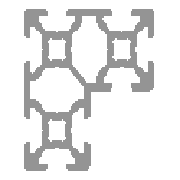
# Autodesk Inventor part: 3 842 992 991-2mm
Saved by Autodesk Inventor 2011 SP1 (Build 150282100, 282)
## iProperties
Created: 2011-02-10
Part Number: 3 842 992 991-2mm
Document SubType Name: Modeling
Designer: S. Wile
Density: 2.71 g/cm^3
Categories: <MemberInstance><Categories><Category DisplayName="Structural Shapes" InternalName="089c4875-fa83-4c05-b084-43b9cc11f5ed" Mnemonic="GRDR"><CategoryParameter DisplayName="Custom Base Point" InternalName="4f1d1b73-316d-484b-a3df-9cbabb16eb77" Mnemonic="shpBasePoint"/><CategoryParameter DisplayName="FG Authored" InternalName="9c666724-f362-4ea7-ac62-f6a007de5c69" Mnemonic="shpFGAuto"/><CategoryParameter DisplayName="Legacy Member ID" InternalName="340afe4f-75d7-48d3-ab7d-943f3c3da468" Mnemonic="LegacyMemberID"/><CategoryParameter DisplayName="Base Length" InternalName="42e34263-8f20-4d0e-ad48-bf1385b87c24" Mnemonic="shplen"/><CategoryParameter DisplayName="Distance of the Center of Gravity X-X" InternalName="26c9bdb8-9c79-4b4f-a92e-8e197583c9c4" Mnemonic="grcendistX"/><CategoryParameter DisplayName="Distance of the Center of Gravity Y-Y" InternalName="bcc4fb17-7af4-436a-8f8c-d0aa3b0248c5" Mnemonic="grcendistY"/><CategoryParameter DisplayName="Torsional Rigidity Modulus" InternalName="26c1ec35-5026-4c63-ad0a-751cf684a536" Mnemonic="torrigmod"/><CategoryParameter DisplayName="Torsional Section Modulus" InternalName="7c55a8dc-8844-49f9-a867-cc677b30ec9a" Mnemonic="torsecmod"/><CategoryParameter DisplayName="Coefficient of Shear Displacement" InternalName="de4c90c6-aaa8-468f-a335-6737b311b5d3" Mnemonic="shdispc"/><CategoryParameter DisplayName="Section Area" InternalName="1ff91680-64b0-4202-b9a3-7fd3f94bba3b" Mnemonic="secarea"/><CategoryParameter DisplayName="Moment of Inertia (x)" InternalName="4cd780bc-73d7-43ac-917a-579e5cbd684d" Mnemonic="inermomx"/><CategoryParameter DisplayName="Moment of Inertia (y)" InternalName="4b9f58ea-bced-460e-81ea-3d29ca5a49e3" Mnemonic="inermomy"/><CategoryParameter DisplayName="Section Module (x)" InternalName="72cfad18-cf51-4ed4-aaa7-c6b224f8419f" Mnemonic="secmodx"/><CategoryParameter DisplayName="Section Module (y)" InternalName="59eaa5e9-d227-48dc-b6c1-6920f96e0f95" Mnemonic="secmody"/><CategoryParameter DisplayName="Radius of Gyration (x)" InternalName="25778675-03e9-40c1-b6a8-4a9ed693320d" Mnemonic="gyrradx"/><CategoryParameter DisplayName="Radius of Gyration (y)" InternalName="bfa18ebe-1636-4dbe-8d42-b263e0b73184" Mnemonic="gyrrady"/><CategoryParameter DisplayName="Shape Thickness" InternalName="d109cf76-8eb4-42fc-9800-4409734adc67" Mnemonic="shpthick"/><CategoryParameter DisplayName="Second Shape Thickness" InternalName="9251a8e1-85fd-4e47-af99-afdb762317d9" Mnemonic="shpthick2"/><CategoryParameter DisplayName="Shape Width" InternalName="7c717d54-a18f-4666-b4d4-573cce22c62c" Mnemonic="shpwdth"/><CategoryParameter DisplayName="Shape Height" InternalName="50274e7d-5ac0-4796-92cb-c59e54983c67" Mnemonic="shpheig"/><CategoryParameter DisplayName="Mass per Length Unit" InternalName="0bb95a10-148f-4027-a459-38d7b056702a" Mnemonic="shpmass"/><CategoryParameter DisplayName="Section Designation" InternalName="5a64d034-428d-49c8-ba32-7619764de20f" Mnemonic="shpdes"/><Category DisplayName="Other" InternalName="f02205ff-2390-476f-921c-0b3185f88e84" Mnemonic="OTHSHP"><CategoryParameter DisplayName="Moment of Inertia (x)" InternalName="ec6737bc-264f-43ed-b0bd-f6d410c2718d" Mnemonic="inermomx"/><CategoryParameter DisplayName="Moment of Inertia (y)" InternalName="044c654e-f649-48ac-84cc-650a29ae31ca" Mnemonic="inermomy"/><CategoryParameter DisplayName="Section Module (x)" InternalName="cac70804-9d39-43bb-be17-56ea1f39a6c2" Mnemonic="secmodx"/><CategoryParameter DisplayName="Section Module (y)" InternalName="88b8bff9-a616-4028-93d5-ed4f79680d13" Mnemonic="secmody"/><CategoryParameter DisplayName="Section Area" InternalName="c46ecdf8-b6eb-4db9-8b25-30258930c1e3" Mnemonic="secarea"/><CategoryParameter DisplayName="Radius of Gyration (x)" InternalName="ee72c61e-565e-4fd6-b448-66e1e1abcb7e" Mnemonic="gyrradx"/><CategoryParameter DisplayName="Radius of Gyration (y)" InternalName="743e1dfe-1bba-408b-b985-cf752b207386" Mnemonic="gyrrady"/><CategoryParameter DisplayName="Shape Thickness" InternalName="12b1a788-9233-48fd-a933-2df8ff42b15f" Mnemonic="shpthick"/><CategoryParameter DisplayName="Mass per Length Unit" InternalName="2fd289d6-9394-4d2d-97e6-6659d7d4551d" Mnemonic="shpmass"/></Category></Category></Categories><FamilyTemplate Id="20x40x40"><FamilyTemplateParameters><FamilyTemplateParameter ObjectType="kUserParameterObject" ValueType="xs:double" Id="1" ObjectReferenceKey="G_L"/><FamilyTemplateParameter ObjectType="kUserParameterObject" ValueType="xs:double" Id="2" ObjectReferenceKey="G_OFFSET_END"/><FamilyTemplateParameter ObjectType="kUserParameterObject" ValueType="xs:double" Id="3" ObjectReferenceKey="G_OFFSET_START"/><FamilyTemplateParameter ObjectType="kUserParameterObject" ValueType="xs:double" Id="4" ObjectReferenceKey="Length"/><FamilyTemplateParameter ObjectType="kPropertyObject" ValueType="xs:string" Id="7" ObjectReferenceKey="{32853F0F-3444-11d1-9E93-0060B03C1CA6}" SubObjectId="52"/><FamilyTemplateParameter ObjectType="kPartComponentDefinitionObject" ValueType="xs:string" Id="8" SubObjectId="Material"/><FamilyTemplateParameter ObjectType="kPropertyObject" ValueType="xs:string" Id="9" ObjectReferenceKey="{32853F0F-3444-11d1-9E93-0060B03C1CA6}" SubObjectId="5"/><FamilyTemplateParameter ObjectType="kPropertyObject" ValueType="xs:string" Id="10" ObjectReferenceKey="{32853F0F-3444-11D1-9E93-0060B03C1CA6}" SubObjectId="55"/><FamilyTemplateParameter ObjectType="kiPartTableColumnObject" ValueType="xs:string" Id="21" ObjectReferenceKey="FILENAME"/><FamilyTemplateParameter ObjectType="kiPartTableColumnObject" ValueType="xs:string" Id="22" ObjectReferenceKey="MEMBER_REVISION"/></FamilyTemplateParameters></FamilyTemplate><CategoryParameterMap><ParamToTemplateMap><ParamToTemplate CategoryParameter="//CategoryParameter[@InternalName='4f1d1b73-316d-484b-a3df-9cbabb16eb77']" ConstantValue="1"/><ParamToTemplate CategoryParameter="//CategoryParameter[@InternalName='9c666724-f362-4ea7-ac62-f6a007de5c69']" ConstantValue="1"/><ParamToTemplate CategoryParameter="//CategoryParameter[@InternalName='2675968c-4ce5-49e0-a4f5-552d29089031']" TemplateParameter="7"/><ParamToTemplate CategoryParameter="//CategoryParameter[@InternalName='8b46a4cc-9585-4fed-90c3-899f57e09a73']" TemplateParameter="21"/><ParamToTemplate CategoryParameter="//CategoryParameter[@InternalName='42e34263-8f20-4d0e-ad48-bf1385b87c24']" TemplateParameter="4"/><ParamToTemplate CategoryParameter="//CategoryParameter[@InternalName='818a152a-d3c3-49ca-80ee-df7d91421b8e']" TemplateParameter="8"/><ParamToTemplate CategoryParameter="//CategoryParameter[@InternalName='a65d44b9-392f-4f4f-857b-e4b3d54996fe']" TemplateParameter="22"/><ParamToTemplate CategoryParameter="//CategoryParameter[@InternalName='016b6077-bfbe-49bd-92c9-d8d59c39c941']" TemplateParameter="9"/></ParamToTemplateMap></CategoryParameterMap></MemberInstance>
Stock Number: 3 842 992 991
Description: PROFILE 20x40x40, -/-
Material: Aluminum-6061
Mass: 2.24182 g
Surface Area: 17.6618 cm^2
Volume: 0.827241 cm^3
Author: S. Wile
Autodesk Inventor part; units mm, degrees
(part 1 of 2)
ref_plane "YZ Plane" through (0, 0, 0) normal (1, 0, 0) x (0, 1, 0)
ref_plane "XZ Plane" through (0, 0, 0) normal (0, 1, 0) x (-1, 0, 0)
ref_plane "XY Plane" through (0, 0, 0) normal (0, 0, 1) x (1, 0, 0)
sketch "20x40x40" plane through (0, 0, 0) normal (0, 0, 1) x (1, 0, 0)
  arc A0 (64.9127, 49.9559) -> (64.8824, 50.1695) centre (64.7308, 50.0391) ccw
  arc A1 (64.9127, 49.9559) -> (64.9127, 47.6687) centre (67.4136, 48.8123) ccw
  arc A2 (55.9136, 39.0445) -> (55.7672, 39.3981) centre (55.4136, 39.0445) ccw
  line L0 (50.9994, 44.1658) -> (55.7672, 39.3981)
  arc A3 (50.9994, 44.1658) -> (50.6458, 44.3123) centre (50.6458, 43.8123) ccw
  line L1 (48.3672, 44.3123) -> (50.6458, 44.3123)
  arc A4 (48.2672, 44.3391) -> (48.3672, 44.3123) centre (48.3672, 44.5123) ccw
  line L2 (47.5136, 44.7742) -> (48.2672, 44.3391)
  arc A5 (47.5136, 44.7742) -> (47.3136, 44.7742) centre (47.4136, 44.601) ccw
  line L3 (46.56, 44.3391) -> (47.3136, 44.7742)
  arc A6 (46.46, 44.3123) -> (46.56, 44.3391) centre (46.46, 44.5123) ccw
  line L4 (44.1814, 44.3123) -> (46.46, 44.3123)
  arc A7 (44.1814, 44.3123) -> (43.8278, 44.1658) centre (44.1814, 43.8123) ccw
  line L5 (43.8278, 44.1658) -> (41.5601, 41.8981)
  arc A8 (40.1458, 41.3123) -> (41.5601, 41.8981) centre (40.1458, 43.3123) ccw
  line L6 (40.1458, 41.3123) -> (39.4136, 41.3123)
  arc A9 (39.4136, 41.3123) -> (38.9136, 40.8123) centre (39.4136, 40.8123) ccw
  line L7 (38.9136, 36.8123) -> (38.9136, 40.8123)
  arc A10 (38.9136, 36.8123) -> (39.4136, 36.3123) centre (39.4136, 36.8123) ccw
  line L8 (40.1458, 36.3123) -> (39.4136, 36.3123)
  arc A11 (41.5601, 35.7265) -> (40.1458, 36.3123) centre (40.1458, 34.3123) ccw
  line L9 (43.8278, 33.4587) -> (41.5601, 35.7265)
  arc A12 (43.8278, 33.4587) -> (44.1814, 33.3123) centre (44.1814, 33.8123) ccw
  line L10 (46.46, 33.3123) -> (44.1814, 33.3123)
  arc A13 (46.56, 33.2855) -> (46.46, 33.3123) centre (46.46, 33.1123) ccw
  line L11 (47.3136, 32.8504) -> (46.56, 33.2855)
  arc A14 (47.3136, 32.8504) -> (47.5136, 32.8504) centre (47.4136, 33.0236) ccw
  line L12 (48.2672, 33.2855) -> (47.5136, 32.8504)
  arc A15 (48.3672, 33.3123) -> (48.2672, 33.2855) centre (48.3672, 33.1123) ccw
  line L13 (50.6458, 33.3123) -> (48.3672, 33.3123)
  arc A16 (50.6458, 33.3123) -> (50.9994, 33.4587) centre (50.6458, 33.8123) ccw
  line L14 (53.2672, 35.7265) -> (50.9994, 33.4587)
  arc A17 (54.6814, 36.3123) -> (53.2672, 35.7265) centre (54.6814, 34.3123) ccw
  line L15 (54.6814, 36.3123) -> (55.4136, 36.3123)
  arc A18 (55.4136, 36.3123) -> (55.9136, 36.8123) centre (55.4136, 36.8123) ccw
  line L16 (49.9395, 50.1746) -> (50.3052, 50.6129)
  arc A19 (50.3052, 50.6129) -> (50.3152, 50.8562) centre (50.1517, 50.741) ccw
  arc A20 (50.3152, 50.8562) -> (49.4575, 51.7138) centre (47.4136, 48.8123) ccw
  arc A21 (49.4575, 51.7138) -> (49.2142, 51.7039) centre (49.3423, 51.5503) ccw
  line L17 (48.7759, 51.3382) -> (49.2142, 51.7039)
  arc A22 (48.5641, 51.3101) -> (48.7759, 51.3382) centre (48.6478, 51.4917) ccw
  arc A23 (48.5641, 51.3101) -> (46.2631, 51.3101) centre (47.4136, 48.8123) ccw
  arc A24 (46.0513, 51.3382) -> (46.2631, 51.3101) centre (46.1795, 51.4917) ccw
  line L18 (46.0513, 51.3382) -> (45.613, 51.7039)
  arc A25 (45.613, 51.7039) -> (45.3697, 51.7138) centre (45.4849, 51.5503) ccw
  arc A26 (45.3697, 51.7138) -> (44.5121, 50.8562) centre (47.4136, 48.8123) ccw
  arc A27 (44.5121, 50.8562) -> (44.5224, 50.6125) centre (44.6756, 50.741) ccw
  line L19 (44.5224, 50.6125) -> (44.8893, 50.1752)
  arc A28 (44.9267, 49.9861) -> (44.8893, 50.1752) centre (44.7361, 50.0466) ccw
  arc A29 (44.9267, 49.9861) -> (44.9165, 47.6603) centre (47.4136, 48.8123) ccw
  arc A30 (44.8893, 47.4494) -> (44.9165, 47.6603) centre (44.7349, 47.5765) ccw
  line L20 (44.5224, 47.0121) -> (44.8893, 47.4494)
  arc A31 (44.5224, 47.0121) -> (44.5121, 46.7684) centre (44.6756, 46.8836) ccw
  arc A32 (44.5121, 46.7684) -> (45.3777, 45.9051) centre (47.4136, 48.8123) ccw
  arc A33 (45.3777, 45.9051) -> (45.621, 45.9158) centre (45.4924, 46.069) ccw
  line L21 (45.621, 45.9158) -> (46.0582, 46.2827)
  arc A34 (46.27, 46.3114) -> (46.0582, 46.2827) centre (46.1868, 46.1295) ccw
  arc A35 (46.27, 46.3114) -> (48.5641, 46.3145) centre (47.4136, 48.8123) ccw
  arc A36 (48.7759, 46.2864) -> (48.5641, 46.3145) centre (48.6478, 46.1329) ccw
  line L22 (48.7759, 46.2864) -> (49.2142, 45.9207)
  arc A37 (49.2142, 45.9207) -> (49.4575, 45.9107) centre (49.3423, 46.0742) ccw
  arc A38 (49.4575, 45.9107) -> (50.3152, 46.7684) centre (47.4136, 48.8123) ccw
  arc A39 (50.3152, 46.7684) -> (50.3052, 47.0117) centre (50.1517, 46.8836) ccw
  line L23 (50.3052, 47.0117) -> (49.9395, 47.45)
  arc A40 (49.9114, 47.6618) -> (49.9395, 47.45) centre (50.093, 47.5781) ccw
  arc A41 (49.9114, 47.6618) -> (49.9114, 49.9628) centre (47.4136, 48.8123) ccw
  line L24 (46.0513, 31.3382) -> (45.613, 31.7039)
  arc A42 (45.613, 31.7039) -> (45.3697, 31.7138) centre (45.4849, 31.5503) ccw
  arc A43 (45.3697, 31.7138) -> (44.5121, 30.8562) centre (47.4136, 28.8123) ccw
  arc A44 (44.5121, 30.8562) -> (44.522, 30.6129) centre (44.6756, 30.741) ccw
  line L25 (44.522, 30.6129) -> (44.8877, 30.1746)
  arc A45 (44.9158, 29.9628) -> (44.8877, 30.1746) centre (44.7342, 30.0464) ccw
  arc A46 (44.9158, 29.9628) -> (44.9158, 27.6618) centre (47.4136, 28.8123) ccw
  arc A47 (44.8877, 27.45) -> (44.9158, 27.6618) centre (44.7342, 27.5781) ccw
  line L26 (44.522, 27.0117) -> (44.8877, 27.45)
  arc A48 (44.522, 27.0117) -> (44.5121, 26.7684) centre (44.6756, 26.8836) ccw
  arc A49 (44.5121, 26.7684) -> (45.3697, 25.9107) centre (47.4136, 28.8123) ccw
  arc A50 (45.3697, 25.9107) -> (45.613, 25.9207) centre (45.4849, 26.0742) ccw
  line L27 (45.613, 25.9207) -> (46.0513, 26.2864)
  arc A51 (46.2631, 26.3145) -> (46.0513, 26.2864) centre (46.1795, 26.1329) ccw
  arc A52 (46.2631, 26.3145) -> (48.5641, 26.3145) centre (47.4136, 28.8123) ccw
  arc A53 (48.7759, 26.2864) -> (48.5641, 26.3145) centre (48.6478, 26.1329) ccw
  line L28 (48.7759, 26.2864) -> (49.2142, 25.9207)
  arc A54 (49.2142, 25.9207) -> (49.4575, 25.9107) centre (49.3423, 26.0742) ccw
  arc A55 (49.4575, 25.9107) -> (50.3152, 26.7684) centre (47.4136, 28.8123) ccw
  arc A56 (50.3152, 26.7684) -> (50.3052, 27.0117) centre (50.1517, 26.8836) ccw
  line L29 (50.3052, 27.0117) -> (49.9395, 27.45)
  arc A57 (49.9114, 27.6618) -> (49.9395, 27.45) centre (50.093, 27.5781) ccw
  arc A58 (49.9114, 27.6618) -> (49.9114, 29.9628) centre (47.4136, 28.8123) ccw
  arc A59 (49.9395, 30.1746) -> (49.9114, 29.9628) centre (50.093, 30.0464) ccw
  arc A60 (43.8636, 58.6123) -> (43.6636, 58.8123) centre (43.6636, 58.6123) ccw
  line L30 (59.4136, 57.3123) -> (55.4136, 57.3123)
  arc A61 (64.8824, 47.4551) -> (64.9127, 47.6687) centre (64.7308, 47.5855) ccw
  line L31 (55.9136, 36.8123) -> (55.9136, 39.0445)
  arc A62 (49.9395, 50.1746) -> (49.9114, 49.9628) centre (50.093, 50.0464) ccw
  arc A63 (46.0513, 31.3382) -> (46.2631, 31.3101) centre (46.1795, 31.4917) ccw
  arc A64 (55.4136, 57.3123) -> (54.9136, 56.8123) centre (55.4136, 56.8123) ccw
  line L32 (54.9136, 56.0801) -> (54.9136, 56.8123)
  arc A65 (54.3278, 54.6658) -> (54.9136, 56.0801) centre (52.9136, 56.0801) ccw
  line L33 (52.0601, 52.3981) -> (54.3278, 54.6658)
  arc A66 (52.0601, 52.3981) -> (51.9136, 52.0445) centre (52.4136, 52.0445) ccw
  line L34 (51.9136, 49.7659) -> (51.9136, 52.0445)
  arc A67 (51.8868, 49.6659) -> (51.9136, 49.7659) centre (51.7136, 49.7659) ccw
  line L35 (51.4517, 48.9123) -> (51.8868, 49.6659)
  arc A68 (51.4517, 48.9123) -> (51.4517, 48.7123) centre (51.6249, 48.8123) ccw
  line L36 (51.8868, 47.9587) -> (51.4517, 48.7123)
  arc A69 (51.9136, 47.8587) -> (51.8868, 47.9587) centre (51.7136, 47.8587) ccw
  line L37 (51.9136, 45.5801) -> (51.9136, 47.8587)
  arc A70 (51.9136, 45.5801) -> (52.0601, 45.2265) centre (52.4136, 45.5801) ccw
  line L38 (56.8278, 40.4587) -> (52.0601, 45.2265)
  arc A71 (56.8278, 40.4587) -> (57.1814, 40.3123) centre (57.1814, 40.8123) ccw
  line L39 (59.4136, 40.3123) -> (57.1814, 40.3123)
  arc A72 (59.4136, 40.3123) -> (59.9136, 40.8123) centre (59.4136, 40.8123) ccw
  line L40 (59.9136, 41.5445) -> (59.9136, 40.8123)
  arc A73 (60.4994, 42.9587) -> (59.9136, 41.5445) centre (61.9136, 41.5445) ccw
  line L41 (60.4994, 42.9587) -> (62.7672, 45.2265)
  arc A74 (62.7672, 45.2265) -> (62.9136, 45.5801) centre (62.4136, 45.5801) ccw
  line L42 (62.9136, 45.5801) -> (62.9136, 47.8587)
  arc A75 (62.9404, 47.9587) -> (62.9136, 47.8587) centre (63.1136, 47.8587) ccw
  line L43 (62.9404, 47.9587) -> (63.3755, 48.7123)
  arc A76 (63.3755, 48.7123) -> (63.3755, 48.9123) centre (63.2023, 48.8123) ccw
  line L44 (63.3755, 48.9123) -> (62.9404, 49.6659)
  arc A77 (62.9136, 49.7659) -> (62.9404, 49.6659) centre (63.1136, 49.7659) ccw
  line L45 (62.9136, 49.7659) -> (62.9136, 52.0445)
  arc A78 (62.9136, 52.0445) -> (62.7672, 52.3981) centre (62.4136, 52.0445) ccw
  line L46 (62.7672, 52.3981) -> (60.4994, 54.6658)
  arc A79 (59.9136, 56.0801) -> (60.4994, 54.6658) centre (61.9136, 56.0801) ccw
  line L47 (59.9136, 56.0801) -> (59.9136, 56.8123)
  arc A80 (59.9136, 56.8123) -> (59.4136, 57.3123) centre (59.4136, 56.8123) ccw
  line L48 (64.5224, 47.0121) -> (64.8824, 47.4551)
  arc A81 (64.5224, 47.0121) -> (64.5121, 46.7684) centre (64.6756, 46.8836) ccw
  arc A82 (64.5121, 46.7684) -> (65.3697, 45.9107) centre (67.4136, 48.8123) ccw
  arc A83 (65.3697, 45.9107) -> (65.6134, 45.921) centre (65.4849, 46.0742) ccw
  line L49 (65.6134, 45.921) -> (66.0564, 46.2811)
  arc A84 (66.27, 46.3114) -> (66.0564, 46.2811) centre (66.1868, 46.1295) ccw
  arc A85 (66.27, 46.3114) -> (68.5572, 46.3114) centre (67.4136, 48.8123) ccw
  arc A86 (68.769, 46.2827) -> (68.5572, 46.3114) centre (68.6404, 46.1295) ccw
  line L50 (69.2119, 45.9226) -> (68.769, 46.2827)
  arc A87 (69.2119, 45.9226) -> (69.4575, 45.9107) centre (69.3423, 46.0742) ccw
  arc A88 (69.4575, 45.9107) -> (70.3152, 46.7684) centre (67.4136, 48.8123) ccw
  arc A89 (70.3152, 46.7684) -> (70.3033, 47.014) centre (70.1517, 46.8836) ccw
  line L51 (69.9432, 47.4569) -> (70.3033, 47.014)
  arc A90 (69.9145, 47.6687) -> (69.9432, 47.4569) centre (70.0964, 47.5855) ccw
  arc A91 (69.9145, 47.6687) -> (69.9145, 49.9559) centre (67.4136, 48.8123) ccw
  arc A92 (69.9432, 50.1676) -> (69.9145, 49.9559) centre (70.0964, 50.0391) ccw
  line L52 (69.9432, 50.1676) -> (70.3033, 50.6106)
  arc A93 (70.3033, 50.6106) -> (70.3152, 50.8562) centre (70.1517, 50.741) ccw
  arc A94 (70.3152, 50.8562) -> (69.4575, 51.7138) centre (67.4136, 48.8123) ccw
  arc A95 (69.4575, 51.7138) -> (69.2119, 51.702) centre (69.3423, 51.5503) ccw
  line L53 (68.769, 51.3419) -> (69.2119, 51.702)
  arc A96 (68.5572, 51.3132) -> (68.769, 51.3419) centre (68.6404, 51.4951) ccw
  arc A97 (68.5572, 51.3132) -> (66.27, 51.3132) centre (67.4136, 48.8123) ccw
  arc A98 (66.0564, 51.3435) -> (66.27, 51.3132) centre (66.1868, 51.4951) ccw
  line L54 (65.6134, 51.7035) -> (66.0564, 51.3435)
  arc A99 (65.6134, 51.7035) -> (65.3697, 51.7138) centre (65.4849, 51.5503) ccw
  arc A100 (65.3697, 51.7138) -> (64.5121, 50.8562) centre (67.4136, 48.8123) ccw
  arc A101 (64.5121, 50.8562) -> (64.5224, 50.6125) centre (64.6756, 50.741) ccw
  line L55 (64.8824, 50.1695) -> (64.5224, 50.6125)
  arc A102 (38.4136, 51.8123) -> (38.9136, 52.3123) centre (38.4136, 52.3123) ccw
  line L56 (38.1136, 51.8123) -> (38.4136, 51.8123)
  arc A103 (37.9136, 52.0123) -> (38.1136, 51.8123) centre (38.1136, 52.0123) ccw
  line L57 (37.9136, 52.0123) -> (37.9136, 52.1623)
  arc A104 (37.9136, 52.1623) -> (37.7136, 52.3623) centre (37.7136, 52.1623) ccw
  line L58 (37.6136, 52.3623) -> (37.7136, 52.3623)
  arc A105 (37.4136, 52.5623) -> (37.6136, 52.3623) centre (37.6136, 52.5623) ccw
  line L59 (37.4136, 52.5623) -> (37.4136, 57.3123)
  arc A106 (38.9136, 58.8123) -> (37.4136, 57.3123) centre (38.9136, 57.3123) ccw
  line L60 (38.9136, 58.8123) -> (43.6636, 58.8123)
  line L61 (50.7136, 19.3123) -> (50.6136, 19.3123)
  arc A107 (50.4136, 19.5123) -> (50.6136, 19.3123) centre (50.6136, 19.5123) ccw
  line L62 (50.4136, 19.5123) -> (50.4136, 19.8123)
  arc A108 (50.9136, 20.3123) -> (50.4136, 19.8123) centre (50.9136, 19.8123) ccw
  line L63 (50.9136, 20.3123) -> (52.9136, 20.3123)
  arc A109 (52.9136, 20.3123) -> (53.4136, 20.8123) centre (52.9136, 20.8123) ccw
  line L64 (53.4136, 20.8123) -> (53.4136, 21.5445)
  arc A110 (53.4136, 21.5445) -> (53.2672, 21.8981) centre (52.9136, 21.5445) ccw
  line L65 (53.2672, 21.8981) -> (50.9994, 24.1658)
  arc A111 (50.9994, 24.1658) -> (50.6458, 24.3123) centre (50.6458, 23.8123) ccw
  line L66 (50.6458, 24.3123) -> (48.3672, 24.3123)
  arc A112 (48.2672, 24.3391) -> (48.3672, 24.3123) centre (48.3672, 24.5123) ccw
  line L67 (48.2672, 24.3391) -> (47.5136, 24.7742)
  arc A113 (47.5136, 24.7742) -> (47.3136, 24.7742) centre (47.4136, 24.601) ccw
  line L68 (46.56, 24.3391) -> (47.3136, 24.7742)
  arc A114 (46.46, 24.3123) -> (46.56, 24.3391) centre (46.46, 24.5123) ccw
  line L69 (46.46, 24.3123) -> (44.1814, 24.3123)
  arc A115 (44.1814, 24.3123) -> (43.8278, 24.1658) centre (44.1814, 23.8123) ccw
  line L70 (41.5601, 21.8981) -> (43.8278, 24.1658)
  arc A116 (41.5601, 21.8981) -> (41.4136, 21.5445) centre (41.9136, 21.5445) ccw
  line L71 (41.4136, 20.8123) -> (41.4136, 21.5445)
  arc A117 (41.4136, 20.8123) -> (41.9136, 20.3123) centre (41.9136, 20.8123) ccw
  line L72 (41.9136, 20.3123) -> (43.9136, 20.3123)
  arc A118 (44.4136, 19.8123) -> (43.9136, 20.3123) centre (43.9136, 19.8123) ccw
  line L73 (44.4136, 19.5123) -> (44.4136, 19.8123)
  arc A119 (44.2136, 19.3123) -> (44.4136, 19.5123) centre (44.2136, 19.5123) ccw
  line L74 (44.2136, 19.3123) -> (44.1136, 19.3123)
  arc A120 (44.1136, 19.3123) -> (43.9136, 19.1123) centre (44.1136, 19.1123) ccw
  line L75 (43.9136, 19.0123) -> (43.9136, 19.1123)
  arc A121 (43.7136, 18.8123) -> (43.9136, 19.0123) centre (43.7136, 19.0123) ccw
  line L76 (43.7136, 18.8123) -> (38.9136, 18.8123)
  arc A122 (37.4136, 20.3123) -> (38.9136, 18.8123) centre (38.9136, 20.3123) ccw
  line L77 (37.4136, 20.3123) -> (37.4136, 25.0623)
  arc A123 (37.6136, 25.2623) -> (37.4136, 25.0623) centre (37.6136, 25.0623) ccw
  line L78 (37.6136, 25.2623) -> (37.7136, 25.2623)
  arc A124 (37.7136, 25.2623) -> (37.9136, 25.4623) centre (37.7136, 25.4623) ccw
  line L79 (37.9136, 25.4623) -> (37.9136, 25.6123)
  arc A125 (38.1136, 25.8123) -> (37.9136, 25.6123) centre (38.1136, 25.6123) ccw
  line L80 (38.1136, 25.8123) -> (38.4136, 25.8123)
  arc A126 (38.9136, 25.3123) -> (38.4136, 25.8123) centre (38.4136, 25.3123) ccw
  line L81 (38.9136, 25.3123) -> (38.9136, 23.3123)
  arc A127 (38.9136, 23.3123) -> (39.4136, 22.8123) centre (39.4136, 23.3123) ccw
  line L82 (39.4136, 22.8123) -> (40.1458, 22.8123)
  arc A128 (40.1458, 22.8123) -> (40.4994, 22.9587) centre (40.1458, 23.3123) ccw
  line L83 (40.4994, 22.9587) -> (42.7672, 25.2265)
  arc A129 (42.7672, 25.2265) -> (42.9136, 25.5801) centre (42.4136, 25.5801) ccw
  line L84 (42.9136, 25.5801) -> (42.9136, 27.8587)
  arc A130 (42.9404, 27.9587) -> (42.9136, 27.8587) centre (43.1136, 27.8587) ccw
  line L85 (42.9404, 27.9587) -> (43.3755, 28.7123)
  arc A131 (43.3755, 28.7123) -> (43.3755, 28.9123) centre (43.2023, 28.8123) ccw
  line L86 (43.3755, 28.9123) -> (42.9404, 29.6659)
  arc A132 (42.9136, 29.7659) -> (42.9404, 29.6659) centre (43.1136, 29.7659) ccw
  line L87 (42.9136, 29.7659) -> (42.9136, 32.0445)
  arc A133 (42.9136, 32.0445) -> (42.7672, 32.3981) centre (42.4136, 32.0445) ccw
  line L88 (42.7672, 32.3981) -> (40.4994, 34.6658)
  arc A134 (40.4994, 34.6658) -> (40.1458, 34.8123) centre (40.1458, 34.3123) ccw
  line L89 (40.1458, 34.8123) -> (39.4136, 34.8123)
  arc A135 (39.4136, 34.8123) -> (38.9136, 34.3123) centre (39.4136, 34.3123) ccw
  line L90 (38.9136, 32.3123) -> (38.9136, 34.3123)
  arc A136 (38.4136, 31.8123) -> (38.9136, 32.3123) centre (38.4136, 32.3123) ccw
  line L91 (38.4136, 31.8123) -> (38.1136, 31.8123)
  arc A137 (37.9136, 32.0123) -> (38.1136, 31.8123) centre (38.1136, 32.0123) ccw
  line L92 (37.9136, 32.0123) -> (37.9136, 32.1623)
  arc A138 (37.9136, 32.1623) -> (37.7136, 32.3623) centre (37.7136, 32.1623) ccw
  line L93 (37.7136, 32.3623) -> (37.6136, 32.3623)
  arc A139 (37.4136, 32.5623) -> (37.6136, 32.3623) centre (37.6136, 32.5623) ccw
  line L94 (37.4136, 32.5623) -> (37.4136, 45.0623)
  arc A140 (37.6136, 45.2623) -> (37.4136, 45.0623) centre (37.6136, 45.0623) ccw
  line L95 (37.7136, 45.2623) -> (37.6136, 45.2623)
  arc A141 (37.7136, 45.2623) -> (37.9136, 45.4623) centre (37.7136, 45.4623) ccw
  line L96 (37.9136, 45.4623) -> (37.9136, 45.6123)
  arc A142 (38.1136, 45.8123) -> (37.9136, 45.6123) centre (38.1136, 45.6123) ccw
  line L97 (38.4136, 45.8123) -> (38.1136, 45.8123)
  arc A143 (38.9136, 45.3123) -> (38.4136, 45.8123) centre (38.4136, 45.3123) ccw
  line L98 (38.9136, 43.3123) -> (38.9136, 45.3123)
  arc A144 (38.9136, 43.3123) -> (39.4136, 42.8123) centre (39.4136, 43.3123) ccw
  line L99 (40.1458, 42.8123) -> (39.4136, 42.8123)
  arc A145 (40.1458, 42.8123) -> (40.4994, 42.9587) centre (40.1458, 43.3123) ccw
  line L100 (40.4994, 42.9587) -> (42.7672, 45.2265)
  arc A146 (42.7672, 45.2265) -> (42.9136, 45.58) centre (42.4136, 45.58) ccw
  line L101 (42.9136, 45.58) -> (42.9136, 47.8587)
  arc A147 (42.9404, 47.9587) -> (42.9136, 47.8587) centre (43.1136, 47.8587) ccw
  line L102 (42.9404, 47.9587) -> (43.3755, 48.7123)
  arc A148 (43.3755, 48.7123) -> (43.3755, 48.9123) centre (43.2023, 48.8123) ccw
  line L103 (42.9404, 49.6659) -> (43.3755, 48.9123)
  arc A149 (42.9136, 49.7659) -> (42.9404, 49.6659) centre (43.1136, 49.7659) ccw
  line L104 (42.9136, 49.7659) -> (42.9136, 52.0445)
  arc A150 (42.9136, 52.0445) -> (42.7672, 52.3981) centre (42.4136, 52.0445) ccw
  line L105 (40.4994, 54.6658) -> (42.7672, 52.3981)
  arc A151 (40.4994, 54.6658) -> (40.1458, 54.8123) centre (40.1458, 54.3123) ccw
  line L106 (39.4136, 54.8123) -> (40.1458, 54.8123)
  arc A152 (39.4136, 54.8123) -> (38.9136, 54.3123) centre (39.4136, 54.3123) ccw
  line L107 (38.9136, 52.3123) -> (38.9136, 54.3123)
  line L108 (71.4517, 48.7123) -> (71.8868, 47.9587)
  arc A153 (71.9136, 47.8587) -> (71.8868, 47.9587) centre (71.7136, 47.8587) ccw
  line L109 (71.9136, 45.5801) -> (71.9136, 47.8587)
  arc A154 (71.9136, 45.5801) -> (72.0601, 45.2265) centre (72.4136, 45.5801) ccw
  line L110 (72.0601, 45.2265) -> (74.3278, 42.9587)
  arc A155 (74.3278, 42.9587) -> (74.6814, 42.8123) centre (74.6814, 43.3123) ccw
  line L111 (74.6814, 42.8123) -> (75.4136, 42.8123)
  arc A156 (75.4136, 42.8123) -> (75.9136, 43.3123) centre (75.4136, 43.3123) ccw
  line L112 (75.9136, 43.3123) -> (75.9136, 45.3123)
  arc A157 (76.4136, 45.8123) -> (75.9136, 45.3123) centre (76.4136, 45.3123) ccw
  line L113 (76.4136, 45.8123) -> (76.7136, 45.8123)
  arc A158 (76.9136, 45.6123) -> (76.7136, 45.8123) centre (76.7136, 45.6123) ccw
  line L114 (76.9136, 45.5123) -> (76.9136, 45.6123)
  arc A159 (76.9136, 45.5123) -> (77.1136, 45.3123) centre (77.1136, 45.5123) ccw
  line L115 (77.1136, 45.3123) -> (77.2136, 45.3123)
  arc A160 (77.4136, 45.1123) -> (77.2136, 45.3123) centre (77.2136, 45.1123) ccw
  line L116 (77.4136, 40.3123) -> (77.4136, 45.1123)
  arc A161 (75.9136, 38.8123) -> (77.4136, 40.3123) centre (75.9136, 40.3123) ccw
  line L117 (71.1136, 38.8123) -> (75.9136, 38.8123)
  arc A162 (70.9136, 39.0123) -> (71.1136, 38.8123) centre (71.1136, 39.0123) ccw
  line L118 (70.9136, 39.0123) -> (70.9136, 39.1123)
  arc A163 (70.9136, 39.1123) -> (70.7136, 39.3123) centre (70.7136, 39.1123) ccw
  line L119 (70.6136, 39.3123) -> (70.7136, 39.3123)
  arc A164 (70.4136, 39.5123) -> (70.6136, 39.3123) centre (70.6136, 39.5123) ccw
  line L120 (70.4136, 39.5123) -> (70.4136, 39.8123)
  arc A165 (70.9136, 40.3123) -> (70.4136, 39.8123) centre (70.9136, 39.8123) ccw
  line L121 (70.9136, 40.3123) -> (72.9136, 40.3123)
  arc A166 (72.9136, 40.3123) -> (73.4136, 40.8123) centre (72.9136, 40.8123) ccw
  line L122 (73.4136, 40.8123) -> (73.4136, 41.5445)
  arc A167 (73.4136, 41.5445) -> (73.2672, 41.8981) centre (72.9136, 41.5445) ccw
  line L123 (73.2672, 41.8981) -> (70.9994, 44.1658)
  arc A168 (70.9994, 44.1658) -> (70.6458, 44.3123) centre (70.6458, 43.8123) ccw
  line L124 (70.6458, 44.3123) -> (68.3672, 44.3123)
  arc A169 (68.2672, 44.3391) -> (68.3672, 44.3123) centre (68.3672, 44.5123) ccw
  line L125 (68.2672, 44.3391) -> (67.5136, 44.7742)
  arc A170 (67.5136, 44.7742) -> (67.3136, 44.7742) centre (67.4136, 44.601) ccw
  line L126 (66.56, 44.3391) -> (67.3136, 44.7742)
  arc A171 (66.46, 44.3123) -> (66.56, 44.3391) centre (66.46, 44.5123) ccw
  line L127 (66.46, 44.3123) -> (64.1814, 44.3123)
  arc A172 (64.1814, 44.3123) -> (63.8278, 44.1658) centre (64.1814, 43.8123) ccw
  line L128 (61.5601, 41.8981) -> (63.8278, 44.1658)
  arc A173 (61.5601, 41.8981) -> (61.4136, 41.5445) centre (61.9136, 41.5445) ccw
  line L129 (61.4136, 40.8123) -> (61.4136, 41.5445)
  arc A174 (61.4136, 40.8123) -> (61.9136, 40.3123) centre (61.9136, 40.8123) ccw
  line L130 (61.9136, 40.3123) -> (63.9136, 40.3123)
  arc A175 (64.4136, 39.8123) -> (63.9136, 40.3123) centre (63.9136, 39.8123) ccw
  line L131 (64.4136, 39.5123) -> (64.4136, 39.8123)
  arc A176 (64.2136, 39.3123) -> (64.4136, 39.5123) centre (64.2136, 39.5123) ccw
  line L132 (64.0636, 39.3123) -> (64.2136, 39.3123)
  arc A177 (64.0636, 39.3123) -> (63.8636, 39.1123) centre (64.0636, 39.1123) ccw
  line L133 (63.8636, 39.0123) -> (63.8636, 39.1123)
  arc A178 (63.6636, 38.8123) -> (63.8636, 39.0123) centre (63.6636, 39.0123) ccw
  line L134 (58.9136, 38.8123) -> (63.6636, 38.8123)
  arc A179 (58.9136, 38.8123) -> (57.4136, 37.3123) centre (58.9136, 37.3123) ccw
  line L135 (57.4136, 32.5123) -> (57.4136, 37.3123)
  arc A180 (57.2136, 32.3123) -> (57.4136, 32.5123) centre (57.2136, 32.5123) ccw
  line L136 (57.2136, 32.3123) -> (57.1136, 32.3123)
  arc A181 (57.1136, 32.3123) -> (56.9136, 32.1123) centre (57.1136, 32.1123) ccw
  line L137 (56.9136, 32.0123) -> (56.9136, 32.1123)
  arc A182 (56.7136, 31.8123) -> (56.9136, 32.0123) centre (56.7136, 32.0123) ccw
  line L138 (56.7136, 31.8123) -> (56.4136, 31.8123)
  arc A183 (55.9136, 32.3123) -> (56.4136, 31.8123) centre (56.4136, 32.3123) ccw
  line L139 (55.9136, 32.3123) -> (55.9136, 34.3123)
  arc A184 (55.9136, 34.3123) -> (55.4136, 34.8123) centre (55.4136, 34.3123) ccw
  line L140 (54.6814, 34.8123) -> (55.4136, 34.8123)
  arc A185 (54.6814, 34.8123) -> (54.3278, 34.6658) centre (54.6814, 34.3123) ccw
  line L141 (52.0601, 32.3981) -> (54.3278, 34.6658)
  arc A186 (52.0601, 32.3981) -> (51.9136, 32.0445) centre (52.4136, 32.0445) ccw
  line L142 (51.9136, 29.7659) -> (51.9136, 32.0445)
  arc A187 (51.8868, 29.6659) -> (51.9136, 29.7659) centre (51.7136, 29.7659) ccw
  line L143 (51.4517, 28.9123) -> (51.8868, 29.6659)
  arc A188 (51.4517, 28.9123) -> (51.4517, 28.7123) centre (51.6249, 28.8123) ccw
  line L144 (51.4517, 28.7123) -> (51.8868, 27.9587)
  arc A189 (51.9136, 27.8587) -> (51.8868, 27.9587) centre (51.7136, 27.8587) ccw
  line L145 (51.9136, 25.5801) -> (51.9136, 27.8587)
  arc A190 (51.9136, 25.5801) -> (52.0601, 25.2265) centre (52.4136, 25.5801) ccw
  line L146 (52.0601, 25.2265) -> (54.3278, 22.9587)
  arc A191 (54.3278, 22.9587) -> (54.6814, 22.8123) centre (54.6814, 23.3123) ccw
  line L147 (54.6814, 22.8123) -> (55.4136, 22.8123)
  arc A192 (55.4136, 22.8123) -> (55.9136, 23.3123) centre (55.4136, 23.3123) ccw
  line L148 (55.9136, 23.3123) -> (55.9136, 25.3123)
  arc A193 (56.4136, 25.8123) -> (55.9136, 25.3123) centre (56.4136, 25.3123) ccw
  line L149 (56.4136, 25.8123) -> (56.7136, 25.8123)
  arc A194 (56.9136, 25.6123) -> (56.7136, 25.8123) centre (56.7136, 25.6123) ccw
  line L150 (56.9136, 25.5123) -> (56.9136, 25.6123)
  arc A195 (56.9136, 25.5123) -> (57.1136, 25.3123) centre (57.1136, 25.5123) ccw
  line L151 (57.1136, 25.3123) -> (57.2136, 25.3123)
  arc A196 (57.4136, 25.1123) -> (57.2136, 25.3123) centre (57.2136, 25.1123) ccw
  line L152 (57.4136, 20.3123) -> (57.4136, 25.1123)
  arc A197 (55.9136, 18.8123) -> (57.4136, 20.3123) centre (55.9136, 20.3123) ccw
  line L153 (55.9136, 18.8123) -> (51.1136, 18.8123)
  arc A198 (50.9136, 19.0123) -> (51.1136, 18.8123) centre (51.1136, 19.0123) ccw
  line L154 (50.9136, 19.0123) -> (50.9136, 19.1123)
  arc A199 (50.9136, 19.1123) -> (50.7136, 19.3123) centre (50.7136, 19.1123) ccw
  line L155 (49.9395, 30.1746) -> (50.3052, 30.6129)
  arc A200 (50.3052, 30.6129) -> (50.3152, 30.8562) centre (50.1517, 30.741) ccw
  arc A201 (50.3152, 30.8562) -> (49.4575, 31.7138) centre (47.4136, 28.8123) ccw
  arc A202 (49.4575, 31.7138) -> (49.2142, 31.7039) centre (49.3423, 31.5503) ccw
  line L156 (48.7759, 31.3382) -> (49.2142, 31.7039)
  arc A203 (48.5641, 31.3101) -> (48.7759, 31.3382) centre (48.6478, 31.4917) ccw
  arc A204 (48.5641, 31.3101) -> (46.2631, 31.3101) centre (47.4136, 28.8123) ccw
  line L157 (43.8636, 58.5123) -> (43.8636, 58.6123)
  arc A205 (43.8636, 58.5123) -> (44.0636, 58.3123) centre (44.0636, 58.5123) ccw
  line L158 (44.0636, 58.3123) -> (44.2136, 58.3123)
  arc A206 (44.4136, 58.1123) -> (44.2136, 58.3123) centre (44.2136, 58.1123) ccw
  line L159 (44.4136, 57.8123) -> (44.4136, 58.1123)
  arc A207 (43.9136, 57.3123) -> (44.4136, 57.8123) centre (43.9136, 57.8123) ccw
  line L160 (41.9136, 57.3123) -> (43.9136, 57.3123)
  arc A208 (41.9136, 57.3123) -> (41.4136, 56.8123) centre (41.9136, 56.8123) ccw
  line L161 (41.4136, 56.0801) -> (41.4136, 56.8123)
  arc A209 (41.4136, 56.0801) -> (41.5601, 55.7265) centre (41.9136, 56.0801) ccw
  line L162 (43.8278, 53.4587) -> (41.5601, 55.7265)
  arc A210 (43.8278, 53.4587) -> (44.1814, 53.3123) centre (44.1814, 53.8123) ccw
  line L163 (44.1814, 53.3123) -> (46.46, 53.3123)
  arc A211 (46.56, 53.2855) -> (46.46, 53.3123) centre (46.46, 53.1123) ccw
  line L164 (46.56, 53.2855) -> (47.3136, 52.8504)
  arc A212 (47.3136, 52.8504) -> (47.5136, 52.8504) centre (47.4136, 53.0236) ccw
  line L165 (47.5136, 52.8504) -> (48.2672, 53.2855)
  arc A213 (48.3672, 53.3123) -> (48.2672, 53.2855) centre (48.3672, 53.1123) ccw
  line L166 (48.3672, 53.3123) -> (50.6458, 53.3123)
  arc A214 (50.6458, 53.3123) -> (50.9994, 53.4587) centre (50.6458, 53.8123) ccw
  line L167 (50.9994, 53.4587) -> (53.2672, 55.7265)
  arc A215 (53.2672, 55.7265) -> (53.4136, 56.0801) centre (52.9136, 56.0801) ccw
  line L168 (53.4136, 56.0801) -> (53.4136, 56.8123)
  arc A216 (53.4136, 56.8123) -> (52.9136, 57.3123) centre (52.9136, 56.8123) ccw
  line L169 (52.9136, 57.3123) -> (50.9136, 57.3123)
  arc A217 (50.4136, 57.8123) -> (50.9136, 57.3123) centre (50.9136, 57.8123) ccw
  line L170 (50.4136, 57.8123) -> (50.4136, 58.1123)
  arc A218 (50.6136, 58.3123) -> (50.4136, 58.1123) centre (50.6136, 58.1123) ccw
  line L171 (50.6136, 58.3123) -> (50.7136, 58.3123)
  arc A219 (50.7136, 58.3123) -> (50.9136, 58.5123) centre (50.7136, 58.5123) ccw
  line L172 (50.9136, 58.5123) -> (50.9136, 58.6123)
  arc A220 (51.1136, 58.8123) -> (50.9136, 58.6123) centre (51.1136, 58.6123) ccw
  line L173 (51.1136, 58.8123) -> (63.6136, 58.8123)
  arc A221 (63.8136, 58.6123) -> (63.6136, 58.8123) centre (63.6136, 58.6123) ccw
  line L174 (63.8136, 58.5123) -> (63.8136, 58.6123)
  arc A222 (63.8136, 58.5123) -> (64.0136, 58.3123) centre (64.0136, 58.5123) ccw
  line L175 (64.0136, 58.3123) -> (64.2136, 58.3123)
  arc A223 (64.4136, 58.1123) -> (64.2136, 58.3123) centre (64.2136, 58.1123) ccw
  line L176 (64.4136, 57.8123) -> (64.4136, 58.1123)
  arc A224 (63.9136, 57.3123) -> (64.4136, 57.8123) centre (63.9136, 57.8123) ccw
  line L177 (61.9136, 57.3123) -> (63.9136, 57.3123)
  arc A225 (61.9136, 57.3123) -> (61.4136, 56.8123) centre (61.9136, 56.8123) ccw
  line L178 (61.4136, 56.0801) -> (61.4136, 56.8123)
  arc A226 (61.4136, 56.0801) -> (61.5601, 55.7265) centre (61.9136, 56.0801) ccw
  line L179 (61.5601, 55.7265) -> (63.8278, 53.4587)
  arc A227 (63.8278, 53.4587) -> (64.1814, 53.3123) centre (64.1814, 53.8123) ccw
  line L180 (64.1814, 53.3123) -> (66.46, 53.3123)
  arc A228 (66.56, 53.2855) -> (66.46, 53.3123) centre (66.46, 53.1123) ccw
  line L181 (66.56, 53.2855) -> (67.3136, 52.8504)
  arc A229 (67.3136, 52.8504) -> (67.5136, 52.8504) centre (67.4136, 53.0236) ccw
  line L182 (67.5136, 52.8504) -> (68.2672, 53.2855)
  arc A230 (68.3672, 53.3123) -> (68.2672, 53.2855) centre (68.3672, 53.1123) ccw
  line L183 (68.3672, 53.3123) -> (70.6458, 53.3123)
  arc A231 (70.6458, 53.3123) -> (70.9994, 53.4587) centre (70.6458, 53.8123) ccw
  line L184 (70.9994, 53.4587) -> (73.2672, 55.7265)
  arc A232 (73.2672, 55.7265) -> (73.4136, 56.0801) centre (72.9136, 56.0801) ccw
  line L185 (73.4136, 56.0801) -> (73.4136, 56.8123)
  arc A233 (73.4136, 56.8123) -> (72.9136, 57.3123) centre (72.9136, 56.8123) ccw
  line L186 (72.9136, 57.3123) -> (70.9136, 57.3123)
  arc A234 (70.4136, 57.8123) -> (70.9136, 57.3123) centre (70.9136, 57.8123) ccw
  line L187 (70.4136, 57.8123) -> (70.4136, 58.1123)
  arc A235 (70.6136, 58.3123) -> (70.4136, 58.1123) centre (70.6136, 58.1123) ccw
  line L188 (70.6136, 58.3123) -> (70.7136, 58.3123)
  arc A236 (70.7136, 58.3123) -> (70.9136, 58.5123) centre (70.7136, 58.5123) ccw
  line L189 (70.9136, 58.5123) -> (70.9136, 58.6123)
  arc A237 (71.1136, 58.8123) -> (70.9136, 58.6123) centre (71.1136, 58.6123) ccw
  line L190 (71.1136, 58.8123) -> (75.9136, 58.8123)
  arc A238 (77.4136, 57.3123) -> (75.9136, 58.8123) centre (75.9136, 57.3123) ccw
  line L191 (77.4136, 52.5123) -> (77.4136, 57.3123)
  arc A239 (77.2136, 52.3123) -> (77.4136, 52.5123) centre (77.2136, 52.5123) ccw
  line L192 (77.1136, 52.3123) -> (77.2136, 52.3123)
  arc A240 (77.1136, 52.3123) -> (76.9136, 52.1123) centre (77.1136, 52.1123) ccw
  line L193 (76.9136, 52.0123) -> (76.9136, 52.1123)
  arc A241 (76.7136, 51.8123) -> (76.9136, 52.0123) centre (76.7136, 52.0123) ccw
  line L194 (76.4136, 51.8123) -> (76.7136, 51.8123)
  arc A242 (75.9136, 52.3123) -> (76.4136, 51.8123) centre (76.4136, 52.3123) ccw
  line L195 (75.9136, 52.3123) -> (75.9136, 54.3123)
  arc A243 (75.9136, 54.3123) -> (75.4136, 54.8123) centre (75.4136, 54.3123) ccw
  line L196 (74.6814, 54.8123) -> (75.4136, 54.8123)
  arc A244 (74.6814, 54.8123) -> (74.3278, 54.6658) centre (74.6814, 54.3123) ccw
  line L197 (72.0601, 52.3981) -> (74.3278, 54.6658)
  arc A245 (72.0601, 52.3981) -> (71.9136, 52.0445) centre (72.4136, 52.0445) ccw
  line L198 (71.9136, 49.7659) -> (71.9136, 52.0445)
  arc A246 (71.8868, 49.6659) -> (71.9136, 49.7659) centre (71.7136, 49.7659) ccw
  line L199 (71.4517, 48.9123) -> (71.8868, 49.6659)
  arc A247 (71.4517, 48.9123) -> (71.4517, 48.7123) centre (71.6249, 48.8123) ccw